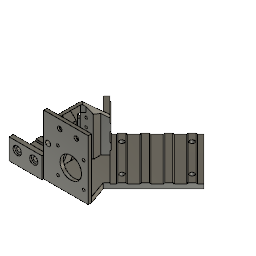
1-Stepper_Mount_Left_V9 (Autodesk Fusion 360 design; units mm, degrees)
Autodesk Fusion 360 part; units mm, degrees
sketch "Main Profile" plane through (0, 0, 0) normal (0, 0, 1) x (1, 0, 0)
  line L0 (-70.4591, -47.4177) -> (-70.4591, -1.8177)
  line L1 (-70.4591, -1.8177) -> (24.3992, 93.0407)
  line L2 (24.3992, 93.0407) -> (76.4989, 40.9411)
  line L3 (76.4989, 40.9411) -> (15.7443, -19.8136)
  line L4 (15.7443, -19.8136) -> (23.3309, -41.4177)
  line L5 (23.3309, -41.4177) -> (23.3309, -45.4177)
  line L6 (23.3309, -45.4177) -> (-30.6591, -45.4177)
  line L7 (-30.6591, -45.4177) -> (-30.6591, -47.4177)
  line L8 (-30.6591, -47.4177) -> (-70.4591, -47.4177)
  line L9 (23.3309, -41.4177) -> (-30.6591, -41.4177)
  line L10 (-30.6591, -41.4177) -> (-30.6591, -45.4177)
  line L11 (-30.6591, -41.4177) -> (-30.6591, -1.8177)
  line L12 (-30.6591, -1.8177) -> (-70.4591, -1.8177)
  line L13 (-32.8483, 28.722) -> (-59.1881, 2.3823)
  line L14 (-59.1881, 2.3823) -> (-27.0147, 2.3823)
  line L15 (-27.0147, 2.3823) -> (-16.7617, 12.6354)
  line L16 (-16.7617, 12.6354) -> (-32.8483, 28.722)
  line L17 (-32.2332, 36.4083) -> (-9.1178, 13.293)
  line L18 (-9.1178, 13.293) -> (-14.7747, 7.6361)
  line L19 (-14.7747, 7.6361) -> (-14.7747, -1.2621)
  line L20 (-27.0147, 2.3823) -> (-30.6591, -1.2621)
  line L21 (-30.6591, -1.2621) -> (-30.6591, -1.8177)
  line L22 (-14.7747, -1.2621) -> (-30.6591, -1.2621)
  line L23 (-26.8991, -41.4177) -> (-26.8991, -4.4883)
  line L24 (-26.8991, -4.4883) -> (-23.6729, -1.2621)
  line L25 (-70.4591, -42.2177) -> (-30.6591, -42.2177)
  line L26 (-26.8991, -16.5877) -> (-20.0991, -16.5877)
  line L27 (-20.0991, -16.5877) -> (-20.0991, -26.4677)
  line L28 (-20.0991, -26.4677) -> (-26.8991, -26.4677)
  line L29 (-26.8991, -26.4677) -> (-26.8991, -16.5877)
  line L30 (-26.8991, -41.4177) -> (-20.0991, -41.4177)
  line L31 (-20.0991, -41.4177) -> (-20.0991, -36.4677)
  line L32 (-20.0991, -36.4677) -> (-26.8991, -36.4677)
  line L33 (-26.8991, -36.4677) -> (-26.8991, -41.4177)
  line L34 (-16.7617, 12.6354) -> (-12.6109, 16.7861)
  line L35 (-32.8483, 28.722) -> (-36.3839, 32.2576)
  line L36 (-9.1178, 13.293) -> (19.8665, -15.6913)
  circle A0 centre (17.8797, 0.5653) radius 5
  circle A1 centre (17.8797, 0.5653) radius 2.75
  circle A2 centre (60.3061, 42.9917) radius 2.75
  circle A3 centre (60.3061, 42.9917) radius 5
  circle A4 centre (-16.0614, 34.5064) radius 2.75
  circle A5 centre (-16.0614, 34.5064) radius 5
  circle A6 centre (26.365, 76.9328) radius 2.75
  circle A7 centre (26.365, 76.9328) radius 5
  circle A8 centre (-60.4591, -31.4177) radius 5
  circle A9 centre (-60.4591, -31.4177) radius 2.75
  circle A10 centre (-40.4591, -31.4177) radius 2.75
  circle A11 centre (-40.4591, -31.4177) radius 5
  circle A12 centre (-60.4591, -11.4177) radius 2.75
  circle A13 centre (-60.4591, -11.4177) radius 5
  circle A14 centre (-40.4591, -11.4177) radius 2.75
  circle A15 centre (-40.4591, -11.4177) radius 5
  dimension "d1" = 45.6
  dimension "d2" = 135
  dimension "d3" = 134.15
  dimension "d4" = 73.68
  dimension "d5" = 85.92
  dimension "d7" = 2
  dimension "d8" = 93.79
  dimension "d9" = 4
  dimension "d10" = 39.8
  dimension "d11" = 4.2
  dimension "d12" = 5
  dimension "d13" = 37.25
  dimension "d14" = 22.75
  dimension "d15" = 8
  dimension "d16" = 32.69
  dimension "d17" = 5.87
  dimension "d18" = 3.76
  dimension "d19" = 40.4
  dimension "d20" = 6.8
  dimension "d21" = 9.88
  dimension "d22" = 4.95
  dimension "d23" = 10
  dimension "d149" = 10
  dimension "d150" = 5.5
  dimension "d153" = -60
  dimension "d154" = -48
  dimension "d155" = 10
  dimension "d156" = 12.9
  dimension "d157" = 10
  dimension "d158" = 5.5
  dimension "d161" = 20
  dimension "d162" = 20
  dimension "d163" = 10
  dimension "d164" = 16
  constraint vertical L0
  constraint perpendicular L1 L2
  constraint perpendicular L2 L3
  constraint vertical L5
  constraint perpendicular L5 L6
  constraint perpendicular L6 L7
  constraint horizontal L8
  constraint perpendicular L7 L9
  constraint perpendicular L6 L10
  constraint perpendicular L9 L11
  constraint horizontal L12
  constraint horizontal L14
  constraint parallel L13 L15
  constraint perpendicular L13 L16
  constraint parallel L1 L13
  constraint coincident L1 L17.start
  constraint perpendicular L1 L17
  constraint perpendicular L17 L18
  constraint vertical L19
  constraint perpendicular L12 L21
  constraint horizontal L22
  constraint collinear L15 L20
  constraint coincident L9 L23.start
  constraint perpendicular L9 L23
  constraint coincident L22 L24.end
  constraint collinear L18 L24
  constraint coincident L0 L25.start
  constraint coincident L10 L25.end
  constraint perpendicular L10 L25
  constraint horizontal L26
  constraint vertical L27
  constraint horizontal L28
  constraint vertical L29
  constraint coincident L23 L26.start
  constraint horizontal L30
  constraint vertical L31
  constraint horizontal L32
  constraint vertical L33
  constraint collinear L27 L31
  constraint coincident L17 L34.end
  constraint perpendicular L17 L34
  constraint coincident L1 L35.end
  constraint perpendicular L1 L35
  constraint coincident L3 L36.end
  constraint perpendicular L3 L36
  constraint concentric A0 A1
  constraint concentric A8 A9
  measures "d1" distance of L0.start L0.end
  measures "d2" angle of L0 L1
  measures "d3" distance of L0.end L1.end
  measures "d4" distance of L1.end L2.end
  measures "d5" distance of L2.end L3.end
  measures "d7" distance of L6 L8
  measures "d8" distance of L0 L5
  measures "d9" distance of L4.end L5.end
  measures "d10" distance of L0.start L7.end
  measures "d11" distance of L12 L14
  measures "d12" distance of L1 L13
  measures "d13" distance of L13.start L13.end
  measures "d14" distance of L13 L15
  measures "d15" distance of L17.end L18.end
  measures "d16" distance of L17.start L17.end
  measures "d17" distance of L16 L17
  measures "d18" distance of L11 L23
  measures "d19" distance of L12 L25
  measures "d20" distance of L23 L27.end
  measures "d21" distance of L26 L28
  measures "d22" distance of L30 L32
  measures "d23" distance of L28 L32
  measures "d149" diameter of A0
  measures "d150" diameter of A1
  measures "d155" distance of L2 A2.centre
  measures "d156" distance of L3 A2.centre
  measures "d157" diameter of A8
  measures "d158" diameter of A9
  measures "d163" distance of L0 A8.centre
  measures "d164" distance of L8 A8.centre
extrude "Extrude1" add sketch "Main Profile" along normal blind 5.35 contours L0 L7 L8 L10 L25 | L0 L10 L11 L12 L25 | L1 L12 L13 L14 L20 L21 L35 | L5 L6 L9 L10 L30 | L1 L16 L17 L34 L35 | L9 L11 L21 L22 L23 L24 L29 L33 | L1 L2 L3 L17 L36 | L13 L14 L15 L16 | L15 L17 L18 L19 L20 L22 L34 | L9 L23 L30 L31 L32 L33 | L3 L4 L9 L18 L19 L22 L23 L24 L26 L27 L28 L31 L32 L36 | L23 L26 L27 L28 L29 | A0 | A1 | A2 | A3 | A4 | A5 | A6 | A7 | A8 | A9 | A10 | A11 | A12 | A13 | A14 | A15 makes body 1
extrude "Extrude7" add sketch "Main Profile" along normal blind 6.5 contours L9 L23 L30 L31 L32 L33 | L3 L4 L9 L18 L19 L22 L23 L24 L26 L27 L28 L31 L32 L36 | L23 L26 L27 L28 L29 bodies 1
extrude "Extrude2" add sketch "Main Profile" along normal blind 72.24 contours L5 L6 L9 L10 L30 bodies 1
extrude "Extrude3" add sketch "Main Profile" along normal blind 59 contours L9 L11 L21 L22 L23 L24 L29 L33 | L15 L17 L18 L19 L20 L22 L34 bodies 1
extrude "Extrude4" add sketch "Main Profile" along normal blind 45.34 contours L1 L16 L17 L34 L35 bodies 1
extrude "Extrude5" add sketch "Main Profile" along normal blind 25.349 contours L0 L7 L8 L10 L25 | L1 L12 L13 L14 L20 L21 L35 bodies 1
chamfer "Chamfer1" distance 23.378 distance2 13.66 1 edges at (-10.8644, 15.0395, 59) measured on face at (-17.7408, 1.704, 59) on bodies 1
extrude "Extrude6" add sketch "Main Profile" along normal up to surface (52.5 mm away) from surface at 6.5 separate body contours L9 L23 L30 L31 L32 L33 | L23 L26 L27 L28 L29 makes body 2 at (-22.3658, -36.4677, 24) makes body 3 at (-26.8991, -23.1744, 24)
chamfer "Chamfer2" distance 6.8 distance2 19.105 2 edges at (-20.0991, -21.5277, 6.5) (-20.0991, -38.9427, 6.5) measured on face at (-24.6325, -23.1744, 6.5) measured on face at (-24.6325, -38.1177, 6.5) on bodies 2 3
chamfer "Chamfer3" distance 19.41 distance2 6.8 1 edges at (-20.0991, -38.9427, 59) measured on face at (-20.0991, -39.7677, 36.7341) on bodies 2
chamfer "Chamfer4" distance 7.095 distance2 6.8 1 edges at (-20.0991, -21.5277, 59) measured on face at (-20.0991, -19.881, 47.8671) on bodies 3
combine "Combine1" operation add target body 1 tool bodies 2 3
sketch "Side A" plane through (-30.6591, 0, 0) normal (-1, 0, 0) x (0, -1, 0)
  line L0 (42.2177, 5.35) -> (42.2177, 25.349)
  line L1 (42.2177, 25.349) -> (45.4177, 25.349)
  line L2 (45.4177, 25.349) -> (45.4177, 72.24)
  line L3 (45.4177, 72.24) -> (41.4177, 72.24)
  line L4 (41.4177, 72.24) -> (41.4177, 59)
  line L5 (41.4177, 59) -> (1.2621, 59)
  line L6 (1.2621, 59) -> (1.2621, 25.349)
  line L7 (1.2621, 25.349) -> (1.8177, 25.349)
  line L8 (1.8177, 25.349) -> (1.8177, 5.35)
  line L9 (1.8177, 5.35) -> (42.2177, 5.35)
  circle A0 centre (31.6177, 15.95) radius 2.6
  circle A1 centre (11.5177, 15.95) radius 2.6
  line L10 (36.3777, 20.97) -> (26.6777, 20.97)
  line L11 (26.6777, 20.97) -> (26.6777, 47.23)
  line L12 (26.6777, 47.23) -> (36.3777, 47.23)
  line L13 (36.3777, 47.23) -> (36.3777, 20.97)
  line L14 (8.1621, 30.05) -> (1.2621, 30.05)
  line L15 (1.2621, 30.05) -> (1.2621, 51.05)
  line L16 (1.2621, 51.05) -> (8.1621, 51.05)
  line L17 (8.1621, 51.05) -> (8.1621, 30.05)
  circle A2 centre (21.5275, 48.0564) radius 1.175
  line L18 (8.6009, 6.65) -> (7.3009, 5.35)
  line L19 (8.6009, 6.65) -> (14.8009, 6.65)
  line L20 (14.8009, 6.65) -> (16.1009, 5.35)
  line L21 (1.8177, 5.35) -> (7.063, 10.5953) construction
  line L22 (3.1177, 12.1332) -> (1.8177, 10.8332)
  line L23 (3.1177, 12.1332) -> (3.1177, 18.3332)
  line L24 (3.1177, 18.3332) -> (1.8177, 19.6332)
  line L25 (22.0177, 5.35) -> (22.0177, 9.5752) construction
  line L26 (35.4344, 6.65) -> (36.7344, 5.35)
  line L27 (35.4344, 6.65) -> (29.2344, 6.65)
  line L28 (29.2344, 6.65) -> (27.9344, 5.35)
  line L29 (40.9177, 12.1332) -> (42.2177, 10.8332)
  line L30 (40.9177, 12.1332) -> (40.9177, 18.3332)
  line L31 (40.9177, 18.3332) -> (42.2177, 19.6332)
  dimension "d47" = 5.2
  dimension "d48" = 10.6
  dimension "d49" = 10.6
  dimension "d52" = -20.1
  dimension "d53" = 0
  dimension "d54" = 9.7
  dimension "d55" = 26.26
  dimension "d56" = 5.84
  dimension "d57" = 15.62
  dimension "d58" = 6.9
  dimension "d59" = 21
  dimension "d60" = 24.7
  dimension "d61" = 2.35
  dimension "d62" = 0.8264
  dimension "d63" = 5.1502
  dimension "d66" = 135
  dimension "d67" = 135
  dimension "d68" = 1.3
  dimension "d69" = 6.2
  dimension "d70" = 5.4832
  dimension "d71" = 45
  constraint horizontal L10
  constraint vertical L11
  constraint horizontal L12
  constraint vertical L13
  constraint horizontal L14
  constraint vertical L15
  constraint horizontal L16
  constraint vertical L17
  constraint coincident L6 L15.end
  constraint coincident L9 L18.end
  constraint parallel L9 L19
  constraint coincident L9 L20.end
  constraint coincident L8.end L9.start
  constraint symmetric L18.start L21 L22.start
  constraint symmetric L18.end L21 L22.end
  constraint symmetric L19.end L21 L23.end
  constraint symmetric L20.end L21 L24.end
  constraint coincident L9 L25.start
  constraint perpendicular L9 L25
  constraint symmetric L18.start L25 L26.start
  constraint symmetric L18.end L25 L26.end
  constraint symmetric L19.end L25 L27.end
  constraint symmetric L20.end L25 L28.end
  constraint symmetric L22.start L25 L29.start
  constraint symmetric L22.end L25 L29.end
  constraint symmetric L23.end L25 L30.end
  constraint symmetric L24.end L25 L31.end
  constraint midpoint L9 L25.start
  measures "d47" diameter of A0
  measures "d48" distance of L0 A0.centre
  measures "d49" distance of L9 A0.centre
  measures "d54" distance of L11 L13
  measures "d55" distance of L10 L12
  measures "d56" distance of L0 L13
  measures "d57" distance of L9 L10
  measures "d58" distance of L15 L17
  measures "d59" distance of L14 L16
  measures "d60" distance of L9 L14
  measures "d61" diameter of A2
  measures "d62" distance of L12 A2.centre
  measures "d63" distance of L11 A2.centre
  measures "d66" angle of L18 L19
  measures "d67" angle of L19 L20
  measures "d68" distance of L9 L19
  measures "d69" distance of L18.start L19.end
  measures "d70" distance of L8 L18.end
  measures "d71" angle of L9 L21
extrude "Extrude8" cut sketch "Side A" against normal blind 18.135 contours L6 L14 L15 L16 L17 | A0 | A1 | L10 L11 L12 L13 | A2 bodies 1
extrude "Extrude9" add sketch "Side A" along normal up to surface (39.8 mm away) contours L0 L29 L30 L31 | L9 L26 L27 L28 | L9 L18 L19 L20 | L8 L22 L23 L24 bodies 1
sketch "Side B" plane through (-34.3207, 34.3207, 0) normal (-0.707107, 0.707107, 0) x (-0.707107, -0.707107, 0)
  line L0 (2.9177, 25.349) -> (2.9177, 45.34)
  line L1 (2.9177, 45.34) -> (-2.9523, 45.34)
  line L2 (-2.9523, 45.34) -> (-2.9523, 5.35)
  line L3 (-2.9523, 5.35) -> (-83.0426, 5.35)
  line L4 (-83.0426, 5.35) -> (-83.0426, 0)
  line L5 (-83.0426, 0) -> (51.1074, 0)
  line L6 (51.1074, 0) -> (51.1074, 5.35)
  line L7 (51.1074, 5.35) -> (51.1074, 10.8332)
  line L8 (51.1074, 10.8332) -> (51.1074, 19.6332)
  line L9 (51.1074, 19.6332) -> (51.1074, 25.349)
  line L10 (51.1074, 25.349) -> (2.9177, 25.349)
  line L11 (-76.5426, 6.45) -> (-69.5426, 6.45)
  line L12 (-69.5426, 6.45) -> (-68.4426, 5.35)
  line L13 (-76.5426, 6.45) -> (-77.6426, 5.35)
  line L14 (-56.5426, 6.45) -> (-57.6426, 5.35)
  line L15 (-56.5426, 6.45) -> (-49.5426, 6.45)
  line L16 (-49.5426, 6.45) -> (-48.4426, 5.35)
  line L17 (-36.5426, 6.45) -> (-37.6426, 5.35)
  line L18 (-36.5426, 6.45) -> (-29.5426, 6.45)
  line L19 (-29.5426, 6.45) -> (-28.4426, 5.35)
  line L20 (-16.5426, 6.45) -> (-17.6426, 5.35)
  line L21 (-16.5426, 6.45) -> (-9.5426, 6.45)
  line L22 (-9.5426, 6.45) -> (-8.4426, 5.35)
  line L23 (-2.9523, 5.35) -> (-29.5711, 31.9689) construction
  line L24 (-4.0523, 38.9403) -> (-2.9523, 40.0403)
  line L25 (-4.0523, 38.9403) -> (-4.0523, 31.9403)
  line L26 (-4.0523, 31.9403) -> (-2.9523, 30.8403)
  line L27 (-4.0523, 18.9403) -> (-2.9523, 20.0403)
  line L28 (-4.0523, 18.9403) -> (-4.0523, 11.9403)
  line L29 (-4.0523, 11.9403) -> (-2.9523, 10.8403)
  dimension "d74" = 45
  dimension "d75" = 45
  dimension "d76" = 7
  dimension "d77" = 1.1
  dimension "d78" = 6.5
  dimension "d81" = 20
  dimension "d82" = 0
  dimension "d83" = 45
  constraint parallel L3 L11
  constraint coincident L3 L12.end
  constraint coincident L3 L13.end
  constraint coincident L2.end L3.start
  constraint symmetric L17.start L23 L24.start
  constraint symmetric L17.end L23 L24.end
  constraint symmetric L18.end L23 L25.end
  constraint symmetric L19.end L23 L26.end
  constraint symmetric L20.start L23 L27.start
  constraint symmetric L20.end L23 L27.end
  constraint symmetric L21.end L23 L28.end
  constraint symmetric L22.end L23 L29.end
  measures "d74" angle of L3 L13
  measures "d75" angle of L3 L12
  measures "d76" distance of L11.start L11.end
  measures "d77" distance of L3 L11
  measures "d78" distance of L4 L11.start
  measures "d83" angle of L3 L23
extrude "Extrude10" add sketch "Side B" against normal up to surface (73.68 mm away) contours L3 L20 L21 L22 | L3 L11 L12 L13 | L3 L17 L18 L19 | L3 L14 L15 L16 bodies 1
extrude "Extrude11" add sketch "Side B" against normal up to surface (32.69 mm away) contours L2 L24 L25 L26 | L2 L27 L28 L29 bodies 1
sketch "Side C" plane through (0, -47.4177, 0) normal (0, -1, 0) x (1, 0, 0)
  line L0 (-70.4591, 0) -> (-30.6591, 0)
  line L1 (-30.6591, 0) -> (-30.6591, 25.349)
  line L2 (-30.6591, 25.349) -> (-70.4591, 25.349)
  line L3 (-70.4591, 25.349) -> (-70.4591, 0)
  circle A0 centre (-60.5091, 15.849) radius 5
  circle A1 centre (-60.5091, 15.849) radius 2.625
  circle A2 centre (-40.5091, 15.849) radius 2.625
  circle A3 centre (-40.5091, 15.849) radius 5
  circle A4 centre (-11.1587, 62.2054) radius 2.7
  circle A5 centre (-11.1587, 62.2054) radius 5.25
  circle A6 centre (8.8413, 62.2054) radius 2.7
  circle A7 centre (8.8413, 62.2054) radius 5.25
  circle A8 centre (-25.2602, 39.9266) radius 3.05
  circle A9 centre (-25.2602, 39.9266) radius 1.5
  circle A10 centre (2.2143, 28.3183) radius 13
  circle A11 centre (-13.2442, 12.7428) radius 1.6
  circle A12 centre (17.7898, 12.8598) radius 1.6
  circle A13 centre (17.6727, 43.8938) radius 1.6
  circle A14 centre (-13.3612, 43.7768) radius 1.6
  dimension "d88" = 10
  dimension "d89" = 5.25
  dimension "d90" = 9.5
  dimension "d91" = 9.95
  dimension "d94" = 20
  dimension "d95" = 0
  dimension "d96" = 5.4
  dimension "d97" = 10.5
  dimension "d100" = 20
  dimension "d101" = 0
  dimension "d102" = 3
  dimension "d103" = 6.1
  dimension "d104" = 26
  dimension "d105" = 3.2
  dimension "d107" = 360
  dimension "d108" = 28.3183
  dimension "d109" = 2.2143
  dimension "d110" = 13.2442
  dimension "d111" = 12.7428
  dimension "d112" = 39.9266
  dimension "d113" = 25.2602
  dimension "d114" = 62.2054
  dimension "d115" = 11.1587
  constraint concentric A0 A1
  constraint concentric A4 A5
  constraint concentric A8 A9
  measures "d88" diameter of A0
  measures "d89" diameter of A1
  measures "d90" distance of L2 A0.centre
  measures "d91" distance of L3 A0.centre
  measures "d96" diameter of A4
  measures "d97" diameter of A5
  measures "d102" diameter of A9
  measures "d103" diameter of A8
  measures "d104" diameter of A10
  measures "d105" diameter of A11
  measures "d108" vertical distance of origin A10.centre
  measures "d109" horizontal distance of origin A10.centre
  measures "d110" horizontal distance of origin A11.centre
  measures "d111" vertical distance of origin A11.centre
  measures "d112" vertical distance of origin A8.centre
  measures "d113" horizontal distance of origin A8.centre
  measures "d114" vertical distance of origin A4.centre
  measures "d115" horizontal distance of origin A4.centre
extrude "Extrude12" cut sketch "Side C" against normal blind 2 contours A0 | A3 bodies 1
extrude "Extrude13" cut sketch "Side C" against normal blind 13.91 contours A1 | A2 | A4 | A6 | A10 | A11 | A12 | A13 | A14 bodies 1
extrude "Extrude14" cut sketch "Side C" against normal blind 33.241 contours A9 bodies 1
extrude "Extrude15" cut sketch "Side C" against normal blind 9.4 contours A8 bodies 1
extrude "Extrude16" cut sketch "Side C" against normal blind 3 from surface at -28 contours A8 bodies 1
chamfer "Chamfer5" distance 1.411 angle 45 1 edges at (-26.8991, -16.4177, 39.9266) on bodies 1
extrude "Extrude24" cut sketch "Side C" along normal blind 2 from surface at -6 contours A5 | A7 bodies 1
sketch "Side D" plane through (-2.0631, -2.0631, 0) normal (-0.707107, -0.707107, 0) x (0.707107, -0.707107, 0)
  line L0 (-43.5368, 25.349) -> (-43.5368, 5.35)
  line L1 (-43.5368, 5.35) -> (-20.7868, 5.35)
  line L2 (-20.7868, 5.35) -> (-20.7868, 45.34)
  line L3 (-20.7868, 45.34) -> (-48.5368, 45.34)
  line L4 (-48.5368, 45.34) -> (-48.5368, 25.349)
  line L5 (-48.5368, 25.349) -> (-43.5368, 25.349)
  circle A0 centre (-35.4854, 35.272) radius 5
  circle A1 centre (-35.4854, 35.272) radius 2.7
  dimension "d143" = 10
  dimension "d144" = 5.4
  constraint concentric A0 A1
  measures "d143" diameter of A0
  measures "d144" diameter of A1
extrude "Extrude20" cut sketch "Side D" against normal blind 10.613 contours A1 bodies 1
extrude "Extrude21" cut sketch "Side D" against normal blind 1.924 contours A0 bodies 1
sketch "Side E" plane through (0, -1.2621, 0) normal (0, -1, 0) x (1, 0, 0)
  line L0 (-14.7747, 6.5) -> (-14.7747, 53.691)
  line L1 (-14.7747, 53.691) -> (-23.6729, 57.3674)
  line L2 (-23.6729, 57.3674) -> (-23.6729, 51.05)
  line L3 (-23.6729, 51.05) -> (-30.6591, 51.05)
  line L4 (-30.6591, 51.05) -> (-30.6591, 30.05)
  line L5 (-30.6591, 30.05) -> (-23.6729, 30.05)
  line L6 (-23.6729, 30.05) -> (-23.6729, 6.5)
  line L7 (-23.6729, 6.5) -> (-14.7747, 6.5)
  circle A0 centre (-23.4091, 45.75) radius 3.25
  circle A1 centre (-23.4091, 45.75) radius 1.5
  circle A2 centre (-23.4091, 35.75) radius 1.5
  circle A3 centre (-23.4091, 35.75) radius 3.25
  line L8 (-30.6591, 51.05) -> (-30.6591, 30.05)
  dimension "d128" = 6.5
  dimension "d129" = 3
  dimension "d132" = 0
  dimension "d133" = -10
  dimension "d134" = 7.25
  dimension "d135" = 45.75
  constraint concentric A0 A1
  measures "d128" diameter of A0
  measures "d129" diameter of A1
  measures "d134" distance of A0.centre L8
  measures "d135" vertical distance of origin A0.centre
extrude "Extrude17" cut sketch "Side E" against normal blind 27.561 contours A2 bodies 1
extrude "Extrude18" cut sketch "Side E" against normal blind 10.318 contours A1 bodies 1
extrude "Extrude19" cut sketch "Side E" against normal blind 8.703 from surface at -3 contours A0 | A3 bodies 1
extrude "Extrude22" cut sketch "Main Profile" along normal blind 23.489 contours A1 | A2 | A4 | A6 | A9 | A10 | A12 | A14 bodies 1
extrude "Extrude23" cut sketch "Main Profile" along normal blind 2 contours A0 | A3 | A5 | A7 | A8 | A11 | A13 | A15 bodies 1
